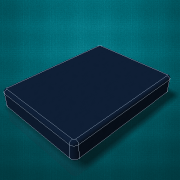
# Autodesk Inventor part: Matress
Saved by Autodesk Inventor 2017 (Build 210142000, 142)
## iProperties
Created: 2017-09-04
Part Number: Matress
Material: Generic
Document SubType Name: Modeling
Designer: Michael
Density: 1 g/cm^3
Appearance: Velvet - Black 1(1)
Author: Michael
Autodesk Inventor part; units mm, degrees
ref_plane "YZ Plane" through (0, 0, 0) normal (1, 0, 0) x (0, 1, 0)
ref_plane "XZ Plane" through (0, 0, 0) normal (0, 1, 0) x (-1, 0, 0)
ref_plane "XY Plane" through (0, 0, 0) normal (0, 0, 1) x (1, 0, 0)
sketch "Sketch1" plane through (0, 0, 0) normal (0, 1, 0) x (-1, 0, 0)
  line L0 (-762, 1016) -> (762, 1016)
  line L1 (762, 1016) -> (762, -1016)
  line L2 (762, -1016) -> (-762, -1016)
  line L3 (-762, -1016) -> (-762, 1016)
  line L4 (-762, 1016) -> (762, -1016) construction
  line L5 (762, 1016) -> (-762, -1016) construction
  point P0 (0, 0)
  dimension "d0" = 1524
  dimension "d1" = 2032
  constraints: 12 end point, 2 midpoint, 2 parallel, 1 horizontal, 1 perpendicular
  measures "d0" distance of L0.start L0.end
  measures "d1" distance of L0.end L1.end
extrude "Extrusion1" add sketch "Sketch1" along normal blind 304.8
fillet "Fillet1" radius 76.2 4 edges at (762, 152.4, 1016) (762, 152.4, -1016) (-762, 152.4, -1016) (-762, 152.4, 1016)
fillet "Fillet2" radius 50.8 8 edges at (739.6815, 304.8, 993.6815) (762, 304.8, 0) (739.6815, 304.8, -993.6815) (0, 304.8, -1016) (-739.6815, 304.8, -993.6815) (-762, 304.8, 0) (-739.6815, 304.8, 993.6815) (0, 304.8, 1016)
fillet "Fillet3" radius 25.4 8 edges at (-739.6815, 0, 993.6815) (-762, 0, 0) (-739.6815, 0, -993.6815) (0, 0, -1016) (739.6815, 0, -993.6815) (762, 0, 0) (739.6815, 0, 993.6815) (0, 0, 1016)
body "Solid1"
